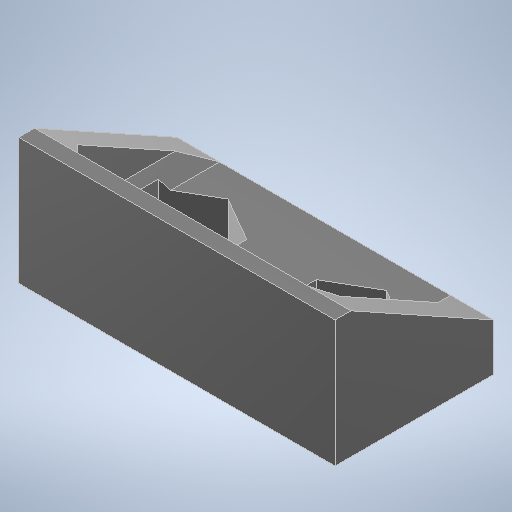
# Autodesk Inventor part: 3D_battery-fix
Saved by Autodesk Inventor 2025.1 (Build 291241020, 241B)
## iProperties
Created: 2024-07-27
Part Number: 3D_battery-fix
Material: 一般
Document SubType Name: Modeling
Designer: 8326d
Density: 1 g/cm^3
Appearance: 滑らか - 黒
Author: 8326d
## iProperties of the stored document 3D_battery-fix_3D プリント.ipt
Created: 2024-09-02
Part Number: 3D_battery-fix_3D プリント
Material: 一般
Document SubType Name: Modeling
Designer: 8326d
Density: 1 g/cm^3
Appearance: 既定
Author: 8326d
Autodesk Inventor part; units mm, degrees
ref_plane "YZ Plane" through (0, 0, 0) normal (1, 0, 0) x (0, 1, 0)
ref_plane "XZ Plane" through (0, 0, 0) normal (0, 1, 0) x (-1, 0, 0)
ref_plane "XY Plane" through (0, 0, 0) normal (0, 0, 1) x (1, 0, 0)
sketch "スケッチ1" plane through (0, 0, 0) normal (1, 0, 0) x (0, 1, 0)
  line L0 (0, 0) -> (3, 0)
  line L1 (3, 0) -> (3, -10)
  line L2 (3, -10) -> (0, -10)
  line L3 (0, -10) -> (0, 0)
  line L4 (3, 0) -> (8, 0)
  line L5 (8, 0) -> (8, -1)
  line L6 (8, -1) -> (3, -1)
  line L7 (3, -1) -> (3, 0)
  line L8 (8, -1) -> (3, -10)
  dimension "d0" = 3
  dimension "d1" = 10
  dimension "d2" = 5
  dimension "d3" = 1
  constraints: 18 end point, 4 parallel, 2 horizontal, 2 perpendicular
  measures "d0" distance of L1.end L2.end
  measures "d1" distance of L0.end L1.end
  measures "d2" distance of L5.end L6.end
  measures "d3" distance of L4.end L5.end
extrude "押し出し1" add sketch "スケッチ1" along normal mid plane 20
sketch "スケッチ2" plane through (0, 0, 0) normal (1, 0, 0) x (0, 1, 0)
  line L0 (3, -10) -> (8, -1) projected
  line L1 (8, -1) -> (3, -1)
  line L2 (3, -1) -> (3, -10)
  line L3 (0, 0) -> (0, -10) projected
  line L4 (8, 0) -> (0, 0) projected
  constraints: 4 end point, 2 parallel, 1 perpendicular
extrude "押し出し2" cut sketch "スケッチ2" along normal mid plane 16.6
sketch "スケッチ3" plane through (-10, 0, -10) normal (0, -1, 0) x (1, 0, 0)
  line L0 (20, 10) -> (20, 0) construction
  line L1 (0, 0) -> (0, 10) construction
  line L2 (20, 5) -> (0, 5) construction
  point P0 (10, 10)
  point P1 (15, 5)
  point P2 (5, 5)
  point P3 (10, 5)
  dimension "d8" = 5
  dimension "d9" = 5
  constraints: 3 midpoint, 2 end point, 2 point on line
  measures "d8" distance of point (15, 5) point (10, 5)
  measures "d9" distance of point (10, 5) point (5, 5)
hole "穴1" at (-5, 0, -5) at (5, 0, -5) direction (0, 1, 0) diameter 3.5 depth 8
sketch "スケッチ4" plane through (-8.3, 3, -10) normal (0, 1, 0) x (1, 0, 0)
  circle A0 centre (13.3, -5) radius 1.75 projected
  circle A1 centre (3.3, -5) radius 1.75 projected
  line L0 (13.3, -1.7668) -> (16.1, -3.3834)
  line L1 (16.1, -3.3834) -> (16.1, -6.6166)
  line L2 (16.1, -6.6166) -> (13.3, -8.2332)
  line L3 (13.3, -8.2332) -> (10.5, -6.6166)
  line L4 (10.5, -6.6166) -> (10.5, -3.3834)
  line L5 (10.5, -3.3834) -> (13.3, -1.7668)
  line L6 (3.3, -1.7668) -> (6.1, -3.3834)
  line L7 (6.1, -3.3834) -> (6.1, -6.6166)
  line L8 (6.1, -6.6166) -> (3.3, -8.2332)
  line L9 (3.3, -8.2332) -> (0.5, -6.6166)
  line L10 (0.5, -6.6166) -> (0.5, -3.3834)
  line L11 (0.5, -3.3834) -> (3.3, -1.7668)
  point P0 (8.3, -10)
  dimension "d17" = 5.6
  dimension "d18" = 5.6
  constraints: 24 end point, 2 coincident, 2 vertical alignment, 26 other
  measures "d17" distance between parallel lines of L1 L4
  measures "d18" distance between parallel lines of L10 L7
extrude "押し出し3" cut sketch "スケッチ4" against normal blind 2.4
chamfer "面取り1" distance 1 angle 45 5 edges at (8.3, 3, -5.5) (-8.3, 3, -5.5) (0, 3, -1) (-8.3, 5.5, -1) (8.3, 5.5, -1)
equation "\"d9\" = d8"
equation "\"d18\" = d17"
